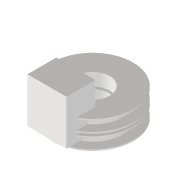
# Autodesk Inventor part: 50_ETL_28by_coil
Saved by Autodesk Inventor 2022 (Build 260153000, 153)
## iProperties
Created: 2021-12-31
Part Number: 50_ETL_28by_coil
Material: Generisch
Document SubType Name: Modeling
Designer: diederichbenedict
Density: 1 g/cm^3
Appearance: Schweißnaht - Messing
Mass: 3.32367 g
Surface Area: 36.1922 cm^2
Volume: 3.32367 cm^3
Author: diederichbenedict
Autodesk Inventor part; units mm, degrees
ref_plane "YZ Plane" through (0, 0, 0) normal (1, 0, 0) x (0, 1, 0)
ref_plane "XZ Plane" through (0, 0, 0) normal (0, 1, 0) x (-1, 0, 0)
ref_plane "XY Plane" through (0, 0, 0) normal (0, 0, 1) x (1, 0, 0)
sketch "Skizze1" plane through (0, 0, 0) normal (0, 0, 1) x (1, 0, 0)
  line L0 (0, 0) -> (-13, 0)
  line L1 (-13, 0) -> (-13, -0.46)
  line L2 (-13, -0.46) -> (-10, -0.46)
  line L3 (-10, -0.46) -> (-10, -3.62)
  line L4 (-10, -3.62) -> (-13, -3.62)
  line L5 (-13, -3.62) -> (-13, -4.08)
  line L6 (-13, -4.08) -> (0, -4.08)
  line L7 (0, -4.08) -> (0, 0)
  line L8 (0, -4.825) -> (-13, -4.825)
  line L9 (-13, -4.825) -> (-13, -5.285)
  line L10 (-13, -5.285) -> (-10, -5.285)
  line L11 (-10, -5.285) -> (-10, -8.445)
  line L12 (-10, -8.445) -> (-13, -8.445)
  line L13 (-13, -8.445) -> (-13, -8.905)
  line L14 (-13, -8.905) -> (0, -8.905)
  line L15 (0, -8.905) -> (0, -4.825)
  dimension "d0" = 13
  dimension "d1" = 0.46
  dimension "d2" = 3
  dimension "d3" = 3.16
  dimension "d4" = 0.46
  dimension "d7" = 4.825
  constraints: 32 end point, 6 perpendicular, 4 point on line, 1 collinear, 1 horizontal, 1 vertical, 15 other
  measures "d0" distance of L0.start L0.end
  measures "d1" distance of L0.end L1.end
  measures "d2" distance of L1.end L2.end
  measures "d3" distance of L2.end L3.end
  measures "d4" distance of L4.end L5.end
  measures "d7" distance of L0.start L8.start
revolve "Umdrehung1" add sketch "Skizze1" angle 360 about axis through (0, -8.905, 0) along (0, 1, 0)
sketch "Skizze2" plane through (0, 0, 0) normal (0, 1, 0) x (1, 0, 0)
  line L0 (6.25, -14.6) -> (-6.25, -14.6)
  line L1 (-6.25, -14.6) -> (-6.25, -5.3061)
  line L2 (-6.25, -5.3061) -> (6.25, -5.3061)
  line L3 (6.25, -5.3061) -> (6.25, -14.6)
  line L4 (6.25, -14.6) -> (-6.25, -5.3061) construction
  line L5 (-6.25, -14.6) -> (6.25, -5.3061) construction
  point P0 (0, 0)
  point P1 (0, -9.9531)
  dimension "d13" = 12.5
  dimension "d14" = 14.6
  constraints: 12 end point, 2 midpoint, 2 parallel, 1 horizontal, 1 perpendicular
  measures "d13" distance of L1.end L2.end
  measures "d14" distance from line of L0 point (0, 0)
extrude "Extrusion1" add sketch "Skizze2" along normal blind 7.4 and the other way blind 7
sketch "Skizze3" plane through (0, -8.905, 0) normal (0, -1, 0) x (1, 0, 0)
  circle A0 centre (0, 0) radius 13 projected
  circle A1 centre (0, 0) radius 6
  dimension "d19" = 12
  constraints: 1 centre point, 1 coincident
  measures "d19" diameter of A1
extrude "Extrusion2" cut sketch "Skizze3" against normal through all contours A1
